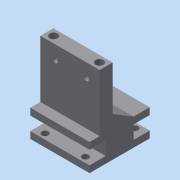
# Autodesk Inventor part: X smooth mount
Saved by Autodesk Inventor 2015 (Build 190159000, 159)
## iProperties
Created: 2016-09-08
Part Number: X smooth mount
Material: Generic
Document SubType Name: Modeling
Designer: Dustin
Density: 1 g/cm^3
Appearance: Default
Author: Dustin
Autodesk Inventor part; units mm, degrees
ref_plane "YZ Plane" through (0, 0, 0) normal (1, 0, 0) x (0, 1, 0)
ref_plane "XZ Plane" through (0, 0, 0) normal (0, 1, 0) x (-1, 0, 0)
sketch "Sketch1" plane through (0, 0, 0) normal (0, 0, 1) x (1, 0, 0)
  line L0 (0, 0) -> (44, 0)
  line L1 (44, 0) -> (44, 9.6635)
  line L2 (44, 9.6635) -> (0, 9.6635)
  line L3 (0, 9.6635) -> (0, 0)
  circle A0 centre (5, 4.8317) radius 3
  circle A1 centre (39, 4.8317) radius 3
  dimension "d0" = 6
  dimension "d1" = 6
  dimension "d2" = 34
  dimension "d3" = 44
  dimension "d4" = 5
  constraints: 8 end point, 2 centre point, 2 parallel, 1 horizontal, 1 perpendicular
  measures "d0" diameter of A0
  measures "d1" diameter of A1
  measures "d2" distance of A1.centre A0.centre
  measures "d3" distance of L1.end L2.end
  measures "d4" distance from line of L3 A0.centre
extrude "Extrusion1" add sketch "Sketch1" along normal blind 42.5
sketch "Sketch2" plane through (0, 9.6635, 0) normal (0, 1, 0) x (1, 0, 0)
  line L0 (44, 0) -> (0, 0) projected
  line L1 (0, 0) -> (0, -42.5) projected
  line L2 (8, -42.5) -> (42, -42.5) projected
  point P0 (11, -32.5)
  point P1 (0, -40.5)
  dimension "d17" = 10
  dimension "d18" = 11
  measures "d17" distance from line of L2 point (11, -32.5)
  measures "d18" distance from line of L1 point (11, -32.5)
hole "Hole1" at (11, 9.6635, 32.5) direction (0, -1, 0) diameter 4 depth 10 tip angle 118
sketch "Sketch3" plane through (0, 9.6635, 0) normal (0, 1, 0) x (1, 0, 0)
  line L0 (8, -42.5) -> (42, -42.5) projected
  line L1 (44, 0) -> (44, -42.5) projected
  point P0 (0, 0)
  point P1 (34, -32.5)
  point P2 (44, -40.5)
  dimension "d19" = 10
  dimension "d20" = 10
  measures "d19" distance from line of L0 point (34, -32.5)
  measures "d20" distance from line of L1 point (34, -32.5)
hole "Hole2" at (34, 9.6635, 32.5) direction (0, -1, 0) diameter 4 depth 10 tip angle 118
sketch "Sketch4" plane through (0, 0, 0) normal (0, 0, -1) x (-1, 0, 0)
  line L0 (0, -7.5) -> (-44, -7.5)
  line L1 (-44, -7.5) -> (-44, 0)
  line L2 (-44, 0) -> (0, 0)
  line L3 (0, 0) -> (0, -7.5)
  line L4 (-44, 9.6635) -> (0, 9.6635)
  line L5 (0, 9.6635) -> (0, 37.1635)
  line L6 (0, 37.1635) -> (-44, 37.1635)
  line L7 (-44, 37.1635) -> (-44, 9.6635)
  circle A0 centre (-39, 4.8317) radius 3 projected
  circle A1 centre (-5, 4.8317) radius 3 projected
  line L8 (0, 0) -> (-44, 0) projected
  line L9 (0, 9.6635) -> (0, 0) projected
  line L10 (-44, 9.6635) -> (0, 9.6635) projected
  line L11 (-44, 0) -> (-44, 9.6635) projected
  dimension "d28" = 7.5
  dimension "d29" = 27.5
  constraints: 16 end point, 4 parallel, 2 horizontal, 2 perpendicular, 1 point on line
  measures "d28" distance of L0.end L1.end
  measures "d29" distance of L6.end L4.start
extrude "Extrusion2" add sketch "Sketch4" along normal blind 20
sketch "Sketch5" plane through (0, 0, -20) normal (0, 0, -1) x (-1, 0, 0)
  arc A0 (-8, 4.8317) -> (-8, 4.8317) centre (-5, 4.8317) ccw projected
  circle A1 centre (-5, 4.8317) radius 3
  circle A2 centre (-39, 4.8317) radius 3 projected
  circle A3 centre (-39, 4.8317) radius 3
  point P0 (0, 0)
  constraints: 2 centre point, 2 coincident
extrude "Extrusion3" add sketch "Sketch5" against normal blind 20
ref_plane "Work Plane2" through (44, 0, 40.5) normal (1, 0, 0) x (0, 0, -1)
sketch "Sketch6" plane through (44, 0, 40.5) normal (1, 0, 0) x (0, 0, -1)
  line L0 (55.5, 37.1635) -> (45.5, 37.1635)
  line L1 (45.5, 37.1635) -> (45.5, 25.1635)
  line L2 (45.5, 25.1635) -> (55.5, 25.1635)
  line L3 (55.5, 25.1635) -> (55.5, 37.1635)
  line L4 (60.5, 37.1635) -> (60.5, -7.5) projected
  line L5 (40.5, -7.5) -> (60.5, -7.5) projected
  line L6 (55.5, -7.5) -> (45.5, -7.5)
  line L7 (45.5, -7.5) -> (45.5, 4.5)
  line L8 (45.5, 4.5) -> (55.5, 4.5)
  line L9 (55.5, 4.5) -> (55.5, -7.5)
  line L10 (40.5, 37.1635) -> (60.5, 37.1635) projected
  point P0 (40.5, 0)
  dimension "d34" = 10
  dimension "d35" = 5
  dimension "d36" = 12
  dimension "d37" = 12
  dimension "d55" = 0
  constraints: 16 end point, 4 parallel, 2 horizontal, 2 perpendicular, 1 point on line
  measures "d34" distance of L0.start L0.end
  measures "d35" distance between parallel lines of L4 L3
  measures "d36" distance of L0.end L1.end
  measures "d37" distance of L6.end L7.end
  measures "d55" distance between parallel lines of L10 L0
extrude "Extrusion4" cut sketch "Sketch6" against normal through all
sketch "Sketch7" plane through (0, 0, -20) normal (0, 0, -1) x (-1, 0, 0)
  line L0 (0, 0) -> (-44, 0) projected
  line L1 (0, 37.1635) -> (-44, 37.1635) projected
  line L2 (-44, -7.5) -> (0, -7.5) projected
  line L3 (0, -7.5) -> (0, 37.1635) projected
  line L4 (-44, 37.1635) -> (-44, -7.5) projected
  point P0 (-37, -3.5)
  point P1 (-7, 33.1635)
  point P2 (-37, 33.1635)
  point P3 (-7, -3.5)
  dimension "d40" = 4
  dimension "d41" = 4
  dimension "d42" = 4
  dimension "d43" = 4
  dimension "d44" = 7
  dimension "d45" = 7
  dimension "d46" = 7
  dimension "d47" = 7
  measures "d40" distance from line of L1 point (-37, 33.163)
  measures "d41" distance from line of L1 point (-7, 33.163)
  measures "d42" distance from line of L2 point (-37, -3.5)
  measures "d43" distance from line of L2 point (-7, -3.5)
  measures "d44" distance from line of L3 point (-7, -3.5)
  measures "d45" distance from line of L3 point (-7, 33.163)
  measures "d46" distance from line of L4 point (-37, 33.163)
  measures "d47" distance from line of L4 point (-37, -3.5)
hole "Hole3" at (37, -3.5, -20) at (7, 33.1635, -20) at (37, 33.1635, -20) at (7, -3.5, -20) direction (0, 0, 1) diameter 4 depth 16 tip angle 118 counterbore diameter 5 counterbore depth 6
sketch "Sketch8" plane through (0, 0, 0) normal (0, 0, 1) x (1, 0, 0)
  line L0 (44, 25.1635) -> (0, 25.1635) projected
  line L1 (0, 9.6635) -> (5, 9.6635)
  line L2 (5, 9.6635) -> (5, 25.1635)
  line L3 (5, 25.1635) -> (0, 25.1635)
  line L4 (0, 25.1635) -> (0, 9.6635)
  point P0 (0, 0)
  dimension "d56" = 5
  constraints: 8 end point, 2 parallel, 1 horizontal, 1 perpendicular, 1 point on line
  measures "d56" distance between parallel lines of L4 L2
extrude "Extrusion5" add sketch "Sketch8" along normal blind 15.5
chamfer "Chamfer1" distance 15.5 angle 45 1 edges at (2.5, 25.1635, 15.5)
sketch "Sketch9" plane through (5, 9.6635, 0) normal (1, 0, 0) x (0, 0, -1)
  line L0 (-15.5, 0) -> (0, 15.5) projected
  line L1 (0, 0) -> (-15.5, 0) projected
  line L2 (0, 15.5) -> (0, 0) projected
  point P0 (0, -9.6635)
extrude "Extrusion6" add sketch "Sketch9" along normal up to surface (39 mm away)
sketch "Sketch11" plane through (44, 0, 42.5) normal (1, 0, 0) x (0, 0, -1)
  line L0 (42.5, 25.1635) -> (33.1498, 9.6635)
  line L1 (33.1498, 9.6635) -> (27, 9.6635)
  line L2 (27, 9.6635) -> (42.5, 25.1635)
  line L3 (42.5, 25.1635) -> (27, 9.6635) projected
  point P0 (42.5, 0)
  constraints: 6 end point, 1 collinear, 1 horizontal
extrude "Extrusion7" cut sketch "Sketch11" against normal through all
body "Solid1"
